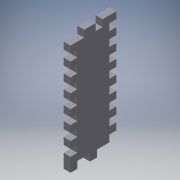
# Autodesk Inventor part: Part2
Saved by Autodesk Inventor 2018 (Build 220112000, 112)
## iProperties
Created: 2018-04-18
Part Number: Part2
Material: Generic
Document SubType Name: Modeling
Designer: Administrator
Density: 1 g/cm^3
Appearance: Default
Author: Administrator
Autodesk Inventor part; units mm, degrees
ref_plane "YZ Plane" through (0, 0, 0) normal (1, 0, 0) x (0, 1, 0)
ref_plane "XZ Plane" through (0, 0, 0) normal (0, 1, 0) x (-1, 0, 0)
ref_plane "XY Plane" through (0, 0, 0) normal (0, 0, 1) x (1, 0, 0)
sketch "Sketch1" plane through (0, 0, 0) normal (0, 1, 0) x (-1, 0, 0)
  line L0 (0, 0) -> (4.7625, 0)
  line L1 (4.7625, 0) -> (4.7625, -31.75)
  line L2 (4.7625, -31.75) -> (0, -31.75)
  line L3 (0, -31.75) -> (0, 0)
  dimension "d0" = 31.75
  dimension "d1" = 4.7625
  constraints: 8 end point, 2 parallel, 1 horizontal, 1 perpendicular
  measures "d0" distance between parallel lines of L2 L0
  measures "d1" distance between parallel lines of L3 L1
extrude "Extrusion1" add sketch "Sketch1" along normal blind 76.2
sketch "Sketch2" plane through (0, 0, 0) normal (0, -1, 0) x (1, 0, 0)
  line L0 (-4.7625, -31.75) -> (-4.7625, 0) projected
  line L1 (0, 0) -> (-4.7625, 0)
  line L2 (-4.7625, 0) -> (-4.7625, -4.7625)
  line L3 (-4.7625, -4.7625) -> (0, -4.7625)
  line L4 (0, -4.7625) -> (0, 0)
  line L5 (0, 0) -> (0, -31.75) projected
  line L6 (0, -13.4938) -> (-4.7625, -13.4938)
  line L7 (-4.7625, -13.4938) -> (-4.7625, -18.2563)
  line L8 (-4.7625, -18.2563) -> (0, -18.2563)
  line L9 (0, -18.2563) -> (0, -13.4938)
  dimension "d4" = 4.7625
  dimension "d5" = 8.7312
  dimension "d6" = 4.7625
  constraints: 16 end point, 4 parallel, 3 point on line, 2 horizontal, 2 perpendicular
  measures "d4" distance between parallel lines of L3 L1
  measures "d5" distance between parallel lines of L3 L6
  measures "d6" distance between parallel lines of L8 L6
extrude "Extrusion2" add sketch "Sketch2" along normal blind 4.7625 contours L0 L6 L5 L8 | L0 L1 L4 L3
sketch "Sketch3" plane through (-4.7625, 76.2, 0) normal (0, 0, 1) x (1, 0, 0)
  line L0 (4.7625, -71.4375) -> (0, -71.4375)
  line L1 (0, -71.4375) -> (0, -66.675)
  line L2 (0, -66.675) -> (4.7625, -66.675)
  line L3 (4.7625, -66.675) -> (4.7625, -71.4375)
  line L4 (4.7625, -80.9625) -> (0, -80.9625) projected
  line L5 (0, -61.9125) -> (4.7625, -61.9125)
  line L6 (4.7625, -61.9125) -> (4.7625, -57.15)
  line L7 (4.7625, -57.15) -> (0, -57.15)
  line L8 (0, -57.15) -> (0, -61.9125)
  line L9 (0, -47.625) -> (4.7625, -47.625)
  line L10 (4.7625, -47.625) -> (4.7625, -52.3875)
  line L11 (4.7625, -52.3875) -> (0, -52.3875)
  line L12 (0, -52.3875) -> (0, -47.625)
  line L13 (0, -38.1) -> (4.7625, -38.1)
  line L14 (4.7625, -38.1) -> (4.7625, -42.8625)
  line L15 (4.7625, -42.8625) -> (0, -42.8625)
  line L16 (0, -42.8625) -> (0, -38.1)
  line L17 (0, -28.575) -> (4.7625, -28.575)
  line L18 (4.7625, -28.575) -> (4.7625, -33.3375)
  line L19 (4.7625, -33.3375) -> (0, -33.3375)
  line L20 (0, -33.3375) -> (0, -28.575)
  line L21 (0, -19.05) -> (4.7625, -19.05)
  line L22 (4.7625, -19.05) -> (4.7625, -23.8125)
  line L23 (4.7625, -23.8125) -> (0, -23.8125)
  line L24 (0, -23.8125) -> (0, -19.05)
  line L25 (0, -9.525) -> (4.7625, -9.525)
  line L26 (4.7625, -9.525) -> (4.7625, -14.2875)
  line L27 (4.7625, -14.2875) -> (0, -14.2875)
  line L28 (0, -14.2875) -> (0, -9.525)
  line L29 (0, 0) -> (4.7625, 0)
  line L30 (4.7625, 0) -> (4.7625, -4.7625)
  line L31 (4.7625, -4.7625) -> (0, -4.7625)
  line L32 (0, -4.7625) -> (0, 0)
  line L33 (4.7625, -80.9625) -> (4.7625, 0) projected
  line L34 (0, 0) -> (4.7625, 0) projected
  line L35 (0, 0) -> (0, -80.9625) projected
  line L36 (4.7625, -80.9625) -> (0, -80.9625) projected
  point P0 (4.7625, -76.2)
  dimension "d9" = 9.525
  dimension "d10" = 4.7625
  dimension "d11" = 4.7625
  dimension "d12" = 4.7625
  dimension "d14" = 4.7625
  dimension "d15" = 4.7625
  dimension "d16" = 4.7625
  dimension "d17" = 4.7625
  dimension "d18" = 4.7625
  dimension "d19" = 4.7625
  dimension "d20" = 4.7625
  dimension "d21" = 4.7625
  dimension "d22" = 4.7625
  dimension "d23" = 4.7625
  dimension "d24" = 4.7625
  dimension "d25" = 4.7625
  dimension "d51" = 0
  dimension "d52" = 0
  dimension "d53" = 0
  dimension "d54" = 0
  dimension "d55" = 0
  constraints: 64 end point, 16 parallel, 8 horizontal, 8 perpendicular, 3 point on line
  measures "d9" distance between parallel lines of L4 L0
  measures "d10" distance between parallel lines of L2 L0
  measures "d11" distance between parallel lines of L5 L2
  measures "d12" distance between parallel lines of L5 L7
  measures "d14" distance between parallel lines of L11 L9
  measures "d15" distance between parallel lines of L15 L9
  measures "d16" distance between parallel lines of L13 L15
  measures "d17" distance between parallel lines of L19 L13
  measures "d18" distance between parallel lines of L17 L19
  measures "d19" distance between parallel lines of L7 L11
  measures "d20" distance between parallel lines of L23 L17
  measures "d21" distance between parallel lines of L21 L23
  measures "d22" distance between parallel lines of L25 L27
  measures "d23" distance between parallel lines of L31 L29
  measures "d24" distance between parallel lines of L21 L27
  measures "d25" distance between parallel lines of L31 L25
  measures "d51" distance between parallel lines of L33 L3
  measures "d52" distance between parallel lines of L33 L6
  measures "d53" distance between parallel lines of L33 L10
  measures "d54" distance between parallel lines of L33 L26
  measures "d55" distance between parallel lines of L33 L30
extrude "Extrusion3" cut sketch "Sketch3" against normal blind 4.7625 contours L0 L1 L2 L3 | L5 L8 L7 L6 | L11 L12 L9 L10 | L15 L16 L13 L14 | L19 L20 L17 L18 | L23 L24 L21 L22 | L27 L28 L25 L26 | L31 L32 L29 L30
sketch "Sketch4" plane through (0, 0, -31.75) normal (0, 0, -1) x (-1, 0, 0)
  line L0 (4.7625, 0) -> (0, 0) projected
  line L1 (4.7625, 0) -> (4.7625, 76.2) projected
  line L2 (0, 0) -> (4.7625, 0)
  line L3 (4.7625, 0) -> (4.7625, 4.7625)
  line L4 (4.7625, 4.7625) -> (0, 4.7625)
  line L5 (0, 4.7625) -> (0, 0)
  line L6 (0, 0) -> (0, 76.2) projected
  line L7 (0, 9.525) -> (4.7625, 9.525)
  line L8 (4.7625, 9.525) -> (4.7625, 14.2875)
  line L9 (4.7625, 14.2875) -> (0, 14.2875)
  line L10 (0, 14.2875) -> (0, 9.525)
  line L11 (0, 19.05) -> (4.7625, 19.05)
  line L12 (4.7625, 19.05) -> (4.7625, 23.8125)
  line L13 (4.7625, 23.8125) -> (0, 23.8125)
  line L14 (0, 23.8125) -> (0, 19.05)
  line L15 (0, 28.575) -> (4.7625, 28.575)
  line L16 (4.7625, 28.575) -> (4.7625, 33.3375)
  line L17 (4.7625, 33.3375) -> (0, 33.3375)
  line L18 (0, 33.3375) -> (0, 28.575)
  line L19 (0, 38.1) -> (4.7625, 38.1)
  line L20 (4.7625, 38.1) -> (4.7625, 42.8625)
  line L21 (4.7625, 42.8625) -> (0, 42.8625)
  line L22 (0, 42.8625) -> (0, 38.1)
  line L23 (0, 47.625) -> (4.7625, 47.625)
  line L24 (4.7625, 47.625) -> (4.7625, 52.3875)
  line L25 (4.7625, 52.3875) -> (0, 52.3875)
  line L26 (0, 52.3875) -> (0, 47.625)
  line L27 (0, 57.15) -> (4.7625, 57.15)
  line L28 (4.7625, 57.15) -> (4.7625, 61.9125)
  line L29 (4.7625, 61.9125) -> (0, 61.9125)
  line L30 (0, 61.9125) -> (0, 57.15)
  line L31 (0, 66.675) -> (4.7625, 66.675)
  line L32 (4.7625, 66.675) -> (4.7625, 71.4375)
  line L33 (4.7625, 71.4375) -> (0, 71.4375)
  line L34 (0, 71.4375) -> (0, 66.675)
  dimension "d28" = 4.7625
  dimension "d29" = 4.7625
  dimension "d30" = 4.7625
  dimension "d31" = 4.7625
  dimension "d32" = 4.7625
  dimension "d33" = 4.7625
  dimension "d34" = 4.7625
  dimension "d35" = 4.7625
  dimension "d36" = 4.7625
  dimension "d37" = 4.7625
  dimension "d38" = 4.7625
  dimension "d39" = 4.7625
  dimension "d40" = 4.7625
  dimension "d41" = 4.7625
  dimension "d42" = 4.7625
  constraints: 64 end point, 16 parallel, 8 horizontal, 8 perpendicular, 7 point on line, 9 other
  measures "d28" distance between parallel lines of L0 L4
  measures "d29" distance between parallel lines of L33 L31
  measures "d30" distance between parallel lines of L27 L29
  measures "d31" distance between parallel lines of L23 L25
  measures "d32" distance between parallel lines of L19 L21
  measures "d33" distance between parallel lines of L15 L17
  measures "d34" distance between parallel lines of L11 L13
  measures "d35" distance between parallel lines of L7 L9
  measures "d36" distance between parallel lines of L7 L4
  measures "d37" distance between parallel lines of L11 L9
  measures "d38" distance between parallel lines of L15 L13
  measures "d39" distance between parallel lines of L17 L19
  measures "d40" distance between parallel lines of L23 L21
  measures "d41" distance between parallel lines of L25 L27
  measures "d42" distance between parallel lines of L31 L29
extrude "Extrusion4" cut sketch "Sketch4" against normal blind 4.7625 contours L0 L5 L4 L1 | L7 L6 L9 L1 | L11 L6 L13 L1 | L15 L6 L17 L1 | L19 L6 L21 L1 | L23 L6 L25 L1 | L27 L6 L29 L1 | L31 L6 L33 L1
sketch "Sketch6" plane through (0, 0, -4.7625) normal (1, 0, 0) x (0, 0, -1)
  line L0 (17.4625, 76.2) -> (12.7, 76.2)
  line L1 (12.7, 76.2) -> (12.7, 71.4375)
  line L2 (12.7, 71.4375) -> (17.4625, 71.4375)
  line L3 (17.4625, 71.4375) -> (17.4625, 76.2)
  line L4 (26.9875, 71.4375) -> (26.9875, 76.2) projected
  line L5 (4.7625, 76.2) -> (0, 76.2)
  line L6 (0, 76.2) -> (0, 71.4375)
  line L7 (0, 71.4375) -> (4.7625, 71.4375)
  line L8 (4.7625, 71.4375) -> (4.7625, 76.2)
  line L9 (0, 76.2) -> (0, 71.4375) projected
  point P0 (-4.7625, 0)
  dimension "d45" = 4.7625
  dimension "d46" = 9.525
  dimension "d47" = 4.7625
  dimension "d58" = 0
  constraints: 16 end point, 4 parallel, 2 horizontal, 2 perpendicular
  measures "d45" distance between parallel lines of L3 L1
  measures "d46" distance between parallel lines of L4 L3
  measures "d47" distance between parallel lines of L6 L8
  measures "d58" distance between parallel lines of L9 L6
extrude "Extrusion5" cut sketch "Sketch6" against normal blind 4.7625
body "Solid1"
